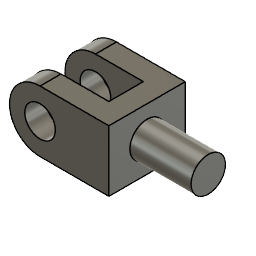
Record 5 (Autodesk Fusion 360 design; units mm, degrees)
part number: 2025-09-30-13-16-28-047
Autodesk Fusion 360 part; units mm, degrees
sketch "Sketch1" plane through (0, 0, 0) normal (0, 0, 1) x (1, 0, 0)
  circle A0 centre (0, 0) radius 8
  line L0 (0, 16) -> (36, 16)
  line L1 (36, 16) -> (36, -16)
  line L2 (36, -16) -> (0, -16)
  arc A1 (0, 16) -> (0, -16) centre (0, 0) ccw
  dimension "d1" = 32
  dimension "d2" = 16
  dimension "d3" = 36
  dimension "d4" = 32
  constraint coincident A0.centre A1.centre
  constraint horizontal L0
  constraint vertical L1
  constraint horizontal L2
  measures "d1" diameter of A1
  measures "d2" diameter of A0
  measures "d3" distance of L0.start L0.end
  measures "d4" distance of L0.start L2.end
extrude "Extrude1" add sketch "Sketch1" along normal blind 40 makes body 1
sketch "Sketch2" plane through (0, 0, 0) normal (1, 0, 0) x (0, 0, -1)
  line L0 (-11, 16) -> (-29, 16)
  line L1 (-29, 16) -> (-29, -16)
  line L2 (-29, -16) -> (-11, -16)
  line L3 (-11, -16) -> (-11, 16)
  line L4 (0, 16) -> (0, -16)
  dimension "d7" = 18
  dimension "d9" = 11
  constraint horizontal L0
  constraint vertical L1
  constraint horizontal L2
  constraint vertical L3
  measures "d7" distance of L0.start L0.end
  measures "d9" distance of L3 L4
extrude "Extrude2" cut sketch "Sketch2" along normal mid plane 76 bodies 1 makes body 2 at (26.6667, 0, 29)
sketch "Sketch3" plane through (36, 0, 0) normal (1, 0, 0) x (0, 0, -1)
  line L0 (-11, 16) -> (-11, -16)
  line L1 (-11, -16) -> (0, -16)
  line L2 (0, -16) -> (0, 16)
  line L3 (0, 16) -> (-11, 16)
  line L4 (-29, 16) -> (-11, 16)
  line L5 (-11, 16) -> (-11, -16)
  line L6 (-11, -16) -> (-29, -16)
  line L7 (-29, -16) -> (-29, 16)
  dimension "d12" = 18
  dimension "d13" = 32
  constraint horizontal L4
  constraint vertical L5
  constraint horizontal L6
  constraint vertical L7
  measures "d12" distance of L4.start L0.start
  measures "d13" distance of L4.start L6.end
extrude "Extrude3" add sketch "Sketch3" against normal blind 11 separate body contours L0 L4 L5 L6 L7 makes body 3
combine "Combine1" operation add target body 3 tool bodies 2 1
sketch "Sketch4" plane through (36, 0, 0) normal (1, 0, 0) x (0, 0, -1)
  line L0 (-40, -16) -> (0, -16)
  line L1 (0, -16) -> (0, 16)
  line L2 (0, 16) -> (-40, 16)
  line L3 (-40, 16) -> (-40, -16)
  circle A0 centre (-20, 0) radius 9
  dimension "d16" = 18
  dimension "d17" = 20
  measures "d16" diameter of A0
  measures "d17" distance of L1 A0.centre
extrude "Extrude4" add sketch "Sketch4" along normal blind 32 separate body contours A0 makes body 4
